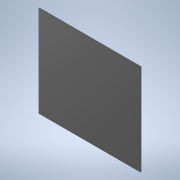
# Autodesk Inventor part: back cover
Saved by Autodesk Inventor 2020.4 (Build 244396000, 396)
## iProperties
Created: 2021-04-08
Part Number: back cover
Material: Wood (Oak)
Document SubType Name: Modeling
Designer: AOB
Mass: 880.627 g
Surface Area: 5879.84 cm^2
Volume: 1158.72 cm^3
Density: 0.76 g/cm^3
Appearance: Smooth - Black
Author: AOB
Autodesk Inventor part; units mm, degrees
ref_plane "YZ Plane" through (0, 0, 0) normal (1, 0, 0) x (0, 1, 0)
ref_plane "XZ Plane" through (0, 0, 0) normal (0, 1, 0) x (-1, 0, 0)
ref_plane "XY Plane" through (0, 0, 0) normal (0, 0, 1) x (1, 0, 0)
sketch "Sketch1" plane through (0, 0, 0) normal (0, 0, 1) x (1, 0, 0)
  line L0 (-8, -5) -> (560, -5)
  line L1 (560, -5) -> (560, -515)
  line L2 (560, -515) -> (-8, -515)
  line L3 (-8, -515) -> (-8, -5)
  point P0 (0, 0)
  dimension "d0" = 568
  dimension "d1" = 510
  constraints: 8 end point, 2 parallel, 1 horizontal, 1 perpendicular
  measures "d0" distance of L1.end L2.end
  measures "d1" distance of L0.end L1.end
extrude "Extrusion1" add sketch "Sketch1" along normal blind 4
body "Solid1"
